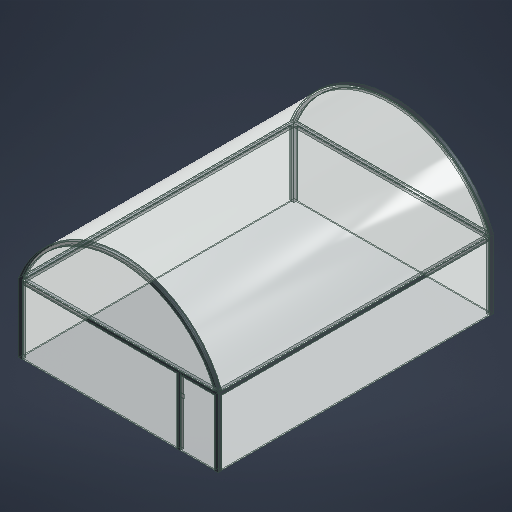
# Autodesk Inventor part: Invernadero
Saved by Autodesk Inventor 2026.1 (Build 301233020, 233B)
## iProperties
Created: 2025-11-02
Part Number: Invernadero
Material: Cristal
Document SubType Name: Modeling
Designer: PAVILION
Density: 2.18 g/cm^3
Appearance: Claro
Author: PAVILION
Autodesk Inventor part; units mm, degrees
note: some values were not read from the file. Chosen so that the rebuilt part matches the saved one: second side of "Extrusión4".
ref_plane "YZ Plane" through (0, 0, 0) normal (1, 0, 0) x (0, 1, 0)
ref_plane "XZ Plane" through (0, 0, 0) normal (0, 1, 0) x (-1, 0, 0)
ref_plane "XY Plane" through (0, 0, 0) normal (0, 0, 1) x (1, 0, 0)
sketch "Boceto1" plane through (0, 0, 0) normal (0, 1, 0) x (-1, 0, 0)
  line L0 (2900, 4000) -> (-2900, 4000)
  line L1 (-2900, 4000) -> (-2900, -4000)
  line L2 (-2900, -4000) -> (2900, -4000)
  line L3 (2900, -4000) -> (2900, 4000)
  line L4 (2900, 4000) -> (-2900, -4000) construction
  line L5 (-2900, 4000) -> (2900, -4000) construction
  point P0 (0, 0)
  dimension "d0" = 8000
  dimension "d1" = 5800
  constraints: 12 end point, 2 midpoint, 2 parallel, 1 horizontal, 1 perpendicular
  measures "d0" distance of L2.end L0.start
  measures "d1" distance of L0.start L0.end
extrude "Extrusión1" add sketch "Boceto1" along normal blind 4000
sketch "Boceto2" plane through (-2900, 0, 4000) normal (0, 0, 1) x (1, 0, 0)
  line L0 (5800, 0) -> (0, 0) projected
  line L1 (5800, 0) -> (5800, 4000) projected
  line L2 (0, 0) -> (5800, 0)
  line L3 (5800, 0) -> (5800, 2000)
  line L4 (5800, 2000) -> (0, 2000)
  line L5 (0, 2000) -> (0, 0)
  arc A0 (5800, 2000) -> (0, 2000) centre (2900, 897.5) ccw
  line L6 (5800, 4000) -> (0, 4000) projected
  line L7 (2900, 4000) -> (0, 4000)
  line L8 (0, 4000) -> (0, 2000)
  line L9 (0, 0) -> (0, 4000) projected
  line L10 (2900, 4000) -> (5800, 4000)
  point P0 (2900, 0)
  dimension "d6" = 3102.5
  constraints: 14 end point, 3 point on circle, 2 parallel, 1 centre point, 1 collinear, 1 horizontal, 1 midpoint, 1 perpendicular
  measures "d6" radius of A0
extrude "Extrusión2" cut sketch "Boceto2" against normal through all contours A0 L6 L1 | L8 L6 A0
shell "Vaciado1" thickness 30 removed faces 1 at (966.6667, 0, -1333.3333)
sketch "Boceto4" plane through (0, 0, 0) normal (0, 1, 0) x (-1, 0, 0)
  line L0 (-2900, 4000) -> (-2800, 4000)
  line L1 (-2800, 4000) -> (-2800, 3900)
  line L2 (-2800, 3900) -> (-2900, 3900)
  line L3 (-2900, 3900) -> (-2900, 4000)
  line L4 (2900, 4000) -> (-2900, 4000) projected
  line L5 (2900, 4000) -> (2800, 4000)
  line L6 (2800, 4000) -> (2800, 3900)
  line L7 (2800, 3900) -> (2900, 3900)
  line L8 (2900, 3900) -> (2900, 4000)
  line L9 (2900, -4000) -> (2900, 4000) projected
  line L10 (2900, -4000) -> (2800, -4000)
  line L11 (2800, -4000) -> (2800, -3900)
  line L12 (2800, -3900) -> (2900, -3900)
  line L13 (2900, -3900) -> (2900, -4000)
  line L14 (-2900, 4000) -> (-2900, -4000) projected
  line L15 (-2900, -4000) -> (-2800, -4000)
  line L16 (-2800, -4000) -> (-2800, -3900)
  line L17 (-2800, -3900) -> (-2900, -3900)
  line L18 (-2900, -3900) -> (-2900, -4000)
  line L19 (2800, -3900) -> (2910, -3900)
  line L20 (2910, -3900) -> (2910, -4010)
  line L21 (2910, -4010) -> (2800, -4010)
  line L22 (2800, -4010) -> (2800, -3900)
  line L23 (-2800, -3900) -> (-2910, -3900)
  line L24 (-2910, -3900) -> (-2910, -4010)
  line L25 (-2910, -4010) -> (-2800, -4010)
  line L26 (-2800, -4010) -> (-2800, -3900)
  line L27 (-2800, 3900) -> (-2910, 3900)
  line L28 (-2910, 3900) -> (-2910, 4010)
  line L29 (-2910, 4010) -> (-2800, 4010)
  line L30 (-2800, 4010) -> (-2800, 3900)
  line L31 (2800, 3900) -> (2910, 3900)
  line L32 (2910, 3900) -> (2910, 4010)
  line L33 (2910, 4010) -> (2800, 4010)
  line L34 (2800, 4010) -> (2800, 3900)
  point P0 (2855, 4010)
  dimension "d16" = 100
  dimension "d17" = 100
  dimension "d18" = 100
  dimension "d19" = 100
  dimension "d20" = 100
  dimension "d21" = 100
  dimension "d22" = 100
  dimension "d23" = 100
  dimension "d26" = 10
  dimension "d27" = 10
  dimension "d28" = 10
  dimension "d29" = 10
  dimension "d30" = 10
  dimension "d31" = 10
  dimension "d32" = 10
  dimension "d33" = 10
  constraints: 64 end point, 16 parallel, 8 horizontal, 8 perpendicular, 1 midpoint
  measures "d16" distance of L0.end L1.end
  measures "d17" distance of L1.end L2.end
  measures "d18" distance of L7.end L4.start
  measures "d19" distance of L6.end L7.end
  measures "d20" distance of L10.end L11.end
  measures "d21" distance of L11.end L12.end
  measures "d22" distance of L15.end L16.end
  measures "d23" distance of L16.end L17.end
  measures "d26" distance between parallel lines of L10 L21
  measures "d27" distance between parallel lines of L20 L13
  measures "d28" distance between parallel lines of L24 L14
  measures "d29" distance between parallel lines of L25 L15
  measures "d30" distance between parallel lines of L28 L14
  measures "d31" distance between parallel lines of L4 L29
  measures "d32" distance from line of L5 point (2855, 4010)
  measures "d33" distance between parallel lines of L32 L9
extrude "Extrusión3" add sketch "Boceto4" along normal blind 2000
sketch "Boceto7" plane through (-2800, 0, 4000) normal (0, 0, 1) x (1, 0, 0)
  line L0 (5710, 0) -> (5710, 2000) projected
  line L1 (-110, 2000) -> (0, 2000) projected
  line L2 (5710, 0) -> (-110, 0)
  line L3 (-110, 0) -> (-110, 2000)
  line L4 (-110, 2000) -> (5710, 2000)
  line L5 (5710, 2000) -> (5710, 0)
  line L6 (5600, 2000) -> (5710, 2000) projected
  arc A0 (5710, 2000) -> (-110, 2000) centre (2800, 897.0748) ccw
  line L7 (5600, 0) -> (5600, 2000) projected
  arc A1 (5600, 2000) -> (0, 2000) centre (2800, 897.0748) ccw
  point P0 (2800, 0)
  dimension "d34" = 3112
  constraints: 8 end point, 4 point on circle, 2 centre point, 2 parallel, 1 concentric, 1 horizontal, 1 perpendicular
  measures "d34" radius of A0
extrude "Extrusión4" add sketch "Boceto7" along normal blind 10 contours L4 A1 L1 A0
sketch "Boceto8" plane through (-2910, 0, 3900) normal (-1, 0, 0) x (0, 0, 1)
  line L0 (0, 2000) -> (110, 2000) projected
  line L1 (110, 0) -> (110, 2000) projected
  line L2 (0, 2000) -> (110, 2000)
  line L3 (110, 2000) -> (110, 1900)
  line L4 (110, 1900) -> (0, 1900)
  line L5 (0, 1900) -> (0, 2000)
  point P0 (-3900, 0)
  dimension "d39" = 100
  constraints: 8 end point, 2 parallel, 1 horizontal, 1 perpendicular, 1 point on line
  measures "d39" distance of L4.end L0.start
extrude "Extrusión5" add sketch "Boceto8" against normal blind 5800
sketch "Boceto9" plane through (2800, 0, -4000) normal (0, 0, -1) x (-1, 0, 0)
  arc A0 (5700, 2000) -> (-100, 2000) centre (2800, 897.5) ccw projected
  arc A1 (5710, 2000) -> (-110, 2000) centre (2800, 897.0748) ccw projected
  line L0 (-67.8825, 2000) -> (5667.8825, 2000) projected
  line L1 (5600, 1900) -> (0, 1900) projected
  arc A2 (5600, 2000) -> (0, 2000) centre (2800, 897.0748) ccw projected
  line L2 (-110, 2000) -> (0, 2000) projected
  line L3 (0, 0) -> (0, 2000) projected
  line L4 (5600, 2000) -> (5710, 2000) projected
  line L5 (5600, 0) -> (5600, 2000) projected
  point P0 (2800, 0)
extrude "Extrusión6" add sketch "Boceto9" along normal blind 10 contours L4 L0 A2 L2 A0 | L5 L1 L3 L0
sketch "Boceto10" plane through (-2870, 0, -3900) normal (0, 0, 1) x (1, 0, 0)
  line L0 (70, 0) -> (70, 2000) projected
  line L1 (-40, 0) -> (-40, 2000) projected
  line L2 (70, 2000) -> (-40, 2000)
  line L3 (-40, 2000) -> (-40, 1900)
  line L4 (-40, 1900) -> (70, 1900)
  line L5 (70, 1900) -> (70, 2000)
  line L6 (15, 1900) -> (15, 2000)
  line L7 (2.1175, 2000) -> (70, 2000) projected
  line L8 (5780, 0) -> (5780, 2000) projected
  line L9 (5670, 0) -> (5670, 2000) projected
  line L10 (5780, 2000) -> (5670, 2000)
  line L11 (5670, 2000) -> (5670, 1900)
  line L12 (5670, 1900) -> (5780, 1900)
  line L13 (5780, 1900) -> (5780, 2000)
  line L14 (5725, 2000) -> (5725, 1900)
  point P0 (2870, 0)
  point P1 (70, 1900)
  dimension "d44" = 100
  dimension "d45" = 100
  constraints: 20 end point, 4 parallel, 3 midpoint, 3 perpendicular, 3 point on line, 2 horizontal
  measures "d44" distance of L6.start L6.end
  measures "d45" distance of L14.start L14.end
extrude "Extrusión7" add sketch "Boceto10" along normal blind 7900
sketch "Boceto11" plane through (2800, 0, -3970) normal (-1, 0, 0) x (0, 0, 1)
  line L0 (-40, 2000) -> (-40, 3906.4674) projected
  line L1 (70, 1900) -> (7870, 1900) projected
  line L2 (-40, 2000) -> (70, 2000)
  line L3 (70, 2000) -> (70, 1900)
  line L4 (70, 1900) -> (-40, 1900)
  line L5 (-40, 1900) -> (-40, 2000)
  point P0 (3970, 0)
  constraints: 8 end point, 2 parallel, 1 horizontal, 1 perpendicular
extrude "Extrusión8" add sketch "Boceto11" along normal up to surface (5710 mm away)
sketch "Boceto15" plane through (0, 897.0748, 4010) normal (0, 0, 1) x (1, 0, 0)
  arc A0 (2910, 1102.9252) -> (-2910, 1102.9252) centre (0, 0) ccw projected
  arc A1 (2800, 1102.9252) -> (-2800, 1102.9252) centre (0, 0) ccw projected
  line L0 (-2800, 1102.9252) -> (2800, 1102.9252) projected
  line L1 (2800, 1102.9252) -> (2910, 1102.9252)
  line L2 (-2800, 1102.9252) -> (-2910, 1102.9252)
  point P0 (0, -897.0748)
  constraints: 4 end point, 2 collinear
extrude "Extrusión12" add sketch "Boceto15" against normal blind 110 contours L1 A1 L2 A0
sketch "Boceto17" plane through (0, 897.5, -4010) normal (0, 0, -1) x (-1, 0, 0)
  arc A0 (2910, 1102.5) -> (-2910, 1102.5) centre (0, -0.4252) ccw projected
  arc A1 (2900, 1102.5) -> (-2900, 1102.5) centre (0, 0) ccw projected
  line L0 (-2910, 1102.5) -> (-2900, 1102.5) projected
  line L1 (2900, 1102.5) -> (2910, 1102.5) projected
  point P0 (0, -897.5)
extrude "Extrusión14" add sketch "Boceto17" against normal blind 110
sketch "Boceto18" plane through (0, 897.5, -3970) normal (0, 0, 1) x (1, 0, 0)
  arc A0 (2800, 1102.5) -> (-2800, 1102.5) centre (0, -0.4252) ccw projected
  arc A1 (2910, 1102.5) -> (-2910, 1102.5) centre (0, -0.4252) ccw projected
  line L0 (2800, 1102.5) -> (-2800, 1102.5) projected
  line L1 (2900, 1102.5) -> (2910, 1102.5) projected
  line L2 (2800, 1102.5) -> (2910, 1102.5)
  line L3 (-2800, 1102.5) -> (-2910, 1102.5)
  point P0 (0, -897.5)
  constraints: 4 end point, 2 horizontal
extrude "Extrusión15" add sketch "Boceto18" along normal blind 70 contours A0 L3 A1 L1 L2
sketch "Boceto19" plane through (-2800, 0, 4000) normal (0, 0, 1) x (1, 0, 0)
  line L0 (0, 1900) -> (5600, 1900) projected
  line L1 (0, 0) -> (5600, 0) projected
  line L2 (5600, 1900) -> (4600, 1900)
  line L3 (4600, 1900) -> (4600, 0)
  line L4 (4600, 0) -> (5600, 0)
  line L5 (5600, 0) -> (5600, 1900)
  line L6 (4600, 0) -> (4500, 0)
  line L7 (4500, 0) -> (4500, 1900)
  line L8 (4500, 1900) -> (4600, 1900)
  line L9 (4600, 1900) -> (4600, 0)
  point P0 (2800, 0)
  dimension "d64" = 100
  dimension "d65" = 1000
  constraints: 16 end point, 4 parallel, 2 horizontal, 2 perpendicular, 2 point on line
  measures "d64" distance between parallel lines of L7 L3
  measures "d65" distance between parallel lines of L3 L5
extrude "Extrusión16" add sketch "Boceto19" along normal blind 10 and the other way blind 100 contours L0 L3 L1 L7
sketch "Boceto20" plane through (2800, 2000, 3900) normal (0, 0, -1) x (-1, 0, 0)
  line L0 (1000, -644.3704) -> (1100, -644.3704)
  line L1 (1100, -644.3704) -> (1100, -749.1876)
  line L2 (1100, -749.1876) -> (1000, -749.1876)
  line L3 (1000, -749.1876) -> (1000, -644.3704)
  line L4 (1000, -100) -> (1000, -2000) projected
  line L5 (1100, -2000) -> (1100, -100) projected
  point P0 (2800, -2000)
  constraints: 8 end point, 2 parallel, 2 point on line, 1 horizontal, 1 perpendicular
extrude "Extrusión17" add sketch "Boceto20" along normal blind 10
